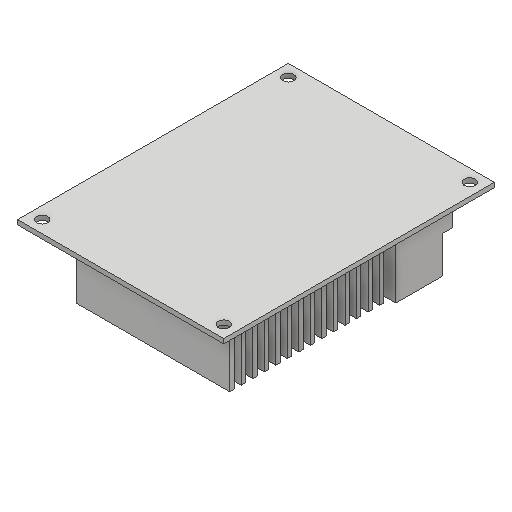
# Autodesk Inventor part: COTS_Generic_MKS_Mosfet_Module_For_Heatbed
Saved by Autodesk Inventor 2026.1 (Build 301233000, 233)
## iProperties
Created: 2017-07-26
Part Number: COTS_Generic_MKS_Mosfet_Module_For_Heatbed
Material: Ogólny
Document SubType Name: Modeling
Designer: Andrzej
Density: 1 g/cm^3
Appearance: Default
Author: Andrzej
Autodesk Inventor part; units mm, degrees
ref_plane "YZ Plane" through (0, 0, 0) normal (1, 0, 0) x (0, 1, 0)
ref_plane "XZ Plane" through (0, 0, 0) normal (0, 1, 0) x (-1, 0, 0)
ref_plane "XY Plane" through (0, 0, 0) normal (0, 0, 1) x (1, 0, 0)
sketch "Szkic1" plane through (0, 0, 0) normal (0, 0, 1) x (1, 0, 0)
  line L0 (-37.6373, 46.6232) -> (29.3627, 46.6232)
  line L1 (29.3627, 46.6232) -> (29.3627, -41.3768)
  line L2 (29.3627, -41.3768) -> (-37.6373, -41.3768)
  line L3 (-37.6373, -41.3768) -> (-37.6373, 46.6232)
  point P0 (0, 0)
  point P1 (-33.6373, 42.6232)
  point P2 (25.3627, 42.6232)
  point P3 (25.3627, -37.3768)
  point P4 (-33.6373, -37.3768)
  dimension "d0" = 88
  dimension "d1" = 67
  dimension "d2" = 59
  dimension "d3" = 80
  dimension "d4" = 80
  dimension "d5" = 59
  dimension "d6" = 4
  dimension "d7" = 4
  dimension "d8" = 4
  dimension "d9" = 4
  dimension "d10" = 4
  dimension "d11" = 4
  dimension "d12" = 4
  constraints: 8 end point, 2 parallel, 1 horizontal, 1 perpendicular
  measures "d0" distance of L2.end L0.start
  measures "d1" distance of L0.start L0.end
  measures "d2" distance of point (25.363, 42.623) point (-33.637, 42.623)
  measures "d3" distance of point (25.363, -37.377) point (25.363, 42.623)
  measures "d4" distance of point (-33.637, 42.623) point (-33.637, -37.377)
  measures "d5" distance of point (25.363, -37.377) point (-33.637, -37.377)
  measures "d6" distance from line of point (-33.637, -37.377) L3
  measures "d7" distance from line of L2 point (-33.637, -37.377)
  measures "d8" distance from line of L3 point (-33.637, 42.623)
  measures "d9" distance from line of L2 point (25.363, -37.377)
  measures "d10" distance from line of L1 point (25.363, -37.377)
  measures "d11" distance from line of L0 point (25.363, 42.623)
  measures "d12" distance from line of L1 point (25.363, 42.623)
extrude "Wyciągnięcie proste1" add sketch "Szkic1" along normal blind 1.5
hole "Otwór1" at (-33.6373, 42.6232, 0) at (25.3627, 42.6232, 0) at (25.3627, -37.3768, 0) at (-33.6373, -37.3768, 0) direction (0, 0, 1) diameter 3.6 end through all
sketch "Szkic2" plane through (0, 0, 0) normal (0, 0, -1) x (-1, 0, 0)
  line L0 (-18.8627, 21.1232) -> (31.1373, 21.1232)
  line L1 (31.1373, 21.1232) -> (31.1373, -28.8768)
  line L2 (31.1373, -28.8768) -> (-18.8627, -28.8768)
  line L3 (-18.8627, -28.8768) -> (-18.8627, 21.1232)
  circle A0 centre (-25.3627, -37.3768) radius 1.8 projected
  circle A1 centre (33.6373, 42.6232) radius 1.8 projected
  circle A2 centre (-25.3627, 42.6232) radius 1.8 projected
  circle A3 centre (33.6373, -37.3768) radius 1.8 projected
  line L4 (37.6373, 46.6232) -> (-29.3627, 46.6232) projected
  line L5 (-29.3627, 46.6232) -> (-29.3627, -41.3768) projected
  line L6 (-29.3627, -41.3768) -> (37.6373, -41.3768) projected
  line L7 (37.6373, -41.3768) -> (37.6373, 46.6232) projected
  line L8 (-16.3627, 42.6232) -> (23.6373, 42.6232)
  line L9 (23.6373, 42.6232) -> (23.6373, 27.6232)
  line L10 (23.6373, 27.6232) -> (-16.3627, 27.6232)
  line L11 (-16.3627, 27.6232) -> (-16.3627, 42.6232)
  point P0 (0, 0)
  dimension "d22" = 50
  dimension "d23" = 50
  dimension "d24" = 6.5
  dimension "d25" = 12.5
  dimension "d26" = 40
  dimension "d27" = 15
  dimension "d28" = 13
  dimension "d29" = 4
  constraints: 16 end point, 4 parallel, 2 horizontal, 2 perpendicular
  measures "d22" distance of L1.end L2.end
  measures "d23" distance of L0.end L1.end
  measures "d24" distance between parallel lines of L7 L1
  measures "d25" distance between parallel lines of L6 L2
  measures "d26" distance of L9.end L10.end
  measures "d27" distance of L8.end L9.end
  measures "d28" distance between parallel lines of L5 L11
  measures "d29" distance between parallel lines of L4 L8
extrude "Wyciągnięcie proste2" add sketch "Szkic2" along normal blind 25 contours L0 L1 L2 L3
sketch "Szkic3" plane through (0, 0, -25) normal (0, 0, -1) x (-1, 0, 0)
  line L0 (31.1373, 21.1232) -> (-18.8627, 21.1232) projected
  line L1 (-18.8627, 21.1232) -> (-18.8627, -28.8768) projected
  line L2 (-18.8627, -28.8768) -> (31.1373, -28.8768) projected
  line L3 (31.1373, -28.8768) -> (31.1373, 21.1232) projected
  line L4 (-18.8627, -28.8768) -> (-18.8627, 21.1232) projected
  line L5 (-18.8627, -27.5268) -> (31.1373, -27.5268)
  line L6 (31.1373, -27.5268) -> (31.1373, -25.1768)
  line L7 (31.1373, -25.1768) -> (-18.8627, -25.1768)
  line L8 (-18.8627, -25.1768) -> (-18.8627, -27.5268)
  line L9 (-18.8627, -23.7768) -> (31.1373, -23.7768)
  line L10 (31.1373, -23.7768) -> (31.1373, -21.4268)
  line L11 (31.1373, -21.4268) -> (-18.8627, -21.4268)
  line L12 (-18.8627, -21.4268) -> (-18.8627, -23.7768)
  line L13 (-18.8627, -20.0268) -> (31.1373, -20.0268)
  line L14 (31.1373, -20.0268) -> (31.1373, -17.6768)
  line L15 (31.1373, -17.6768) -> (-18.8627, -17.6768)
  line L16 (-18.8627, -17.6768) -> (-18.8627, -20.0268)
  line L17 (-18.8627, -16.2768) -> (31.1373, -16.2768)
  line L18 (31.1373, -16.2768) -> (31.1373, -13.9268)
  line L19 (31.1373, -13.9268) -> (-18.8627, -13.9268)
  line L20 (-18.8627, -13.9268) -> (-18.8627, -16.2768)
  line L21 (-18.8627, -12.5268) -> (31.1373, -12.5268)
  line L22 (31.1373, -12.5268) -> (31.1373, -10.1768)
  line L23 (31.1373, -10.1768) -> (-18.8627, -10.1768)
  line L24 (-18.8627, -10.1768) -> (-18.8627, -12.5268)
  line L25 (-18.8627, -8.7768) -> (31.1373, -8.7768)
  line L26 (31.1373, -8.7768) -> (31.1373, -6.4268)
  line L27 (31.1373, -6.4268) -> (-18.8627, -6.4268)
  line L28 (-18.8627, -6.4268) -> (-18.8627, -8.7768)
  line L29 (-18.8627, -5.0268) -> (31.1373, -5.0268)
  line L30 (31.1373, -5.0268) -> (31.1373, -2.6768)
  line L31 (31.1373, -2.6768) -> (-18.8627, -2.6768)
  line L32 (-18.8627, -2.6768) -> (-18.8627, -5.0268)
  line L33 (-18.8627, -1.2768) -> (31.1373, -1.2768)
  line L34 (31.1373, -1.2768) -> (31.1373, 1.0732)
  line L35 (31.1373, 1.0732) -> (-18.8627, 1.0732)
  line L36 (-18.8627, 1.0732) -> (-18.8627, -1.2768)
  line L37 (-18.8627, 2.4732) -> (31.1373, 2.4732)
  line L38 (31.1373, 2.4732) -> (31.1373, 4.8232)
  line L39 (31.1373, 4.8232) -> (-18.8627, 4.8232)
  line L40 (-18.8627, 4.8232) -> (-18.8627, 2.4732)
  line L41 (-18.8627, 6.2232) -> (31.1373, 6.2232)
  line L42 (31.1373, 6.2232) -> (31.1373, 8.5732)
  line L43 (31.1373, 8.5732) -> (-18.8627, 8.5732)
  line L44 (-18.8627, 8.5732) -> (-18.8627, 6.2232)
  line L45 (-18.8627, 9.9732) -> (31.1373, 9.9732)
  line L46 (31.1373, 9.9732) -> (31.1373, 12.3232)
  line L47 (31.1373, 12.3232) -> (-18.8627, 12.3232)
  line L48 (-18.8627, 12.3232) -> (-18.8627, 9.9732)
  line L49 (-18.8627, 13.7232) -> (31.1373, 13.7232)
  line L50 (31.1373, 13.7232) -> (31.1373, 16.0732)
  line L51 (31.1373, 16.0732) -> (-18.8627, 16.0732)
  line L52 (-18.8627, 16.0732) -> (-18.8627, 13.7232)
  line L53 (-18.8627, 17.4732) -> (31.1373, 17.4732)
  line L54 (31.1373, 17.4732) -> (31.1373, 19.8232)
  line L55 (31.1373, 19.8232) -> (-18.8627, 19.8232)
  line L56 (-18.8627, 19.8232) -> (-18.8627, 17.4732)
  point P0 (0, 0)
  dimension "d32" = 50
  dimension "d33" = 2.35
  dimension "d34" = 1.35
  dimension "d37" = 3.75
  constraints: 104 end point, 2 parallel, 1 horizontal, 1 perpendicular, 1 point on line, 1 vertical, 96 other
  measures "d32" distance of L7.end L6.end
  measures "d33" distance of L6.end L5.end
  measures "d34" distance between parallel lines of L2 L5
  measures "d37" distance of L5.start L9.start
extrude "Wyciągnięcie proste3" cut sketch "Szkic3" against normal blind 17 contours L3 L53 L1 L55 | L3 L49 L1 L51 | L3 L45 L1 L47 | L3 L41 L1 L43 | L3 L37 L1 L39 | L3 L33 L1 L35 | L3 L29 L1 L31 | L3 L25 L1 L27 | L3 L21 L1 L23 | L3 L17 L1 L19 | L3 L13 L1 L15 | L3 L9 L1 L11 | L3 L5 L1 L7
sketch "Szkic4" plane through (-31.1373, -28.8768, 0) normal (-1, 0, 0) x (0, 0, 1)
  line L0 (-8, 42.6) -> (-25, 42.6) projected
  line L1 (-25, 41.2) -> (-25, 42.6) projected
  line L2 (-25, 41.2) -> (-8, 41.2) projected
  line L3 (-8, 41.2) -> (-8, 38.85) projected
  line L4 (-8, 38.85) -> (-25, 38.85) projected
  line L5 (-25, 37.45) -> (-25, 38.85) projected
  line L6 (-25, 37.45) -> (-8, 37.45) projected
  line L7 (-8, 37.45) -> (-8, 35.1) projected
  line L8 (-8, 35.1) -> (-25, 35.1) projected
  line L9 (-25, 33.7) -> (-25, 35.1) projected
  line L10 (-25, 33.7) -> (-8, 33.7) projected
  line L11 (-8, 33.7) -> (-8, 31.35) projected
  line L12 (-8, 31.35) -> (-25, 31.35) projected
  line L13 (-25, 29.95) -> (-25, 31.35) projected
  line L14 (-25, 29.95) -> (-8, 29.95) projected
  line L15 (-8, 29.95) -> (-8, 27.6) projected
  line L16 (-8, 27.6) -> (-25, 27.6) projected
  line L17 (-25, 26.2) -> (-25, 27.6) projected
  line L18 (-25, 26.2) -> (-8, 26.2) projected
  line L19 (-8, 26.2) -> (-8, 23.85) projected
  line L20 (-8, 23.85) -> (-25, 23.85) projected
  line L21 (-25, 22.45) -> (-25, 23.85) projected
  line L22 (-25, 22.45) -> (-8, 22.45) projected
  line L23 (-8, 22.45) -> (-8, 20.1) projected
  line L24 (-8, 20.1) -> (-25, 20.1) projected
  line L25 (-25, 18.7) -> (-25, 20.1) projected
  line L26 (-25, 18.7) -> (-8, 18.7) projected
  line L27 (-8, 18.7) -> (-8, 16.35) projected
  line L28 (-8, 16.35) -> (-25, 16.35) projected
  line L29 (-25, 14.95) -> (-25, 16.35) projected
  line L30 (-25, 14.95) -> (-8, 14.95) projected
  line L31 (-8, 14.95) -> (-8, 12.6) projected
  line L32 (-8, 12.6) -> (-25, 12.6) projected
  line L33 (-25, 11.2) -> (-25, 12.6) projected
  line L34 (-25, 11.2) -> (-8, 11.2) projected
  line L35 (-8, 11.2) -> (-8, 8.85) projected
  line L36 (-8, 8.85) -> (-25, 8.85) projected
  line L37 (-25, 7.45) -> (-25, 8.85) projected
  line L38 (-25, 7.45) -> (-8, 7.45) projected
  line L39 (-8, 7.45) -> (-8, 5.1) projected
  line L40 (-8, 5.1) -> (-25, 5.1) projected
  line L41 (-25, 3.7) -> (-25, 5.1) projected
  line L42 (-25, 3.7) -> (-8, 3.7) projected
  line L43 (-8, 3.7) -> (-8, 1.35) projected
  line L44 (-8, 1.35) -> (-25, 1.35) projected
  line L45 (-25, 0) -> (-25, 1.35) projected
  line L46 (0, 0) -> (-25, 0) projected
  line L47 (0, 50) -> (0, 0) projected
  line L48 (0, 50) -> (-25, 50) projected
  line L49 (-25, 48.7) -> (-25, 50) projected
  line L50 (-25, 48.7) -> (-8, 48.7) projected
  line L51 (-8, 48.7) -> (-8, 46.35) projected
  line L52 (-8, 46.35) -> (-25, 46.35) projected
  line L53 (-25, 44.95) -> (-25, 46.35) projected
  line L54 (-25, 44.95) -> (-8, 44.95) projected
  line L55 (-8, 44.95) -> (-8, 42.6) projected
  line L56 (0, 50) -> (0, 0) projected
  line L57 (0, 50) -> (-25, 50) projected
  line L58 (0, 0) -> (-5, 0)
  line L59 (-5, 0) -> (-5, 50)
  line L60 (-5, 50) -> (0, 50)
  line L61 (0, 50) -> (0, 0)
  point P0 (0, 28.8768)
  dimension "d44" = 5
  constraints: 8 end point, 2 parallel, 1 horizontal, 1 perpendicular, 1 point on line
  measures "d44" distance of L59.end L60.end
extrude "Wyciągnięcie proste4" cut sketch "Szkic4" against normal blind 16 contours L48 L47 L46 L59
sketch "Szkic5" plane through (18.8627, -28.8768, 0) normal (1, 0, 0) x (0, 0, -1)
  line L0 (25, 42.6) -> (8, 42.6) projected
  line L1 (8, 42.6) -> (8, 44.95) projected
  line L2 (8, 44.95) -> (25, 44.95) projected
  line L3 (25, 46.35) -> (25, 44.95) projected
  line L4 (25, 46.35) -> (8, 46.35) projected
  line L5 (8, 46.35) -> (8, 48.7) projected
  line L6 (8, 48.7) -> (25, 48.7) projected
  line L7 (25, 50) -> (25, 48.7) projected
  line L8 (0, 50) -> (25, 50) projected
  line L9 (0, 0) -> (0, 50) projected
  line L10 (0, 0) -> (25, 0) projected
  line L11 (25, 1.35) -> (25, 0) projected
  line L12 (25, 1.35) -> (8, 1.35) projected
  line L13 (8, 1.35) -> (8, 3.7) projected
  line L14 (8, 3.7) -> (25, 3.7) projected
  line L15 (25, 5.1) -> (25, 3.7) projected
  line L16 (25, 5.1) -> (8, 5.1) projected
  line L17 (8, 5.1) -> (8, 7.45) projected
  line L18 (8, 7.45) -> (25, 7.45) projected
  line L19 (25, 8.85) -> (25, 7.45) projected
  line L20 (25, 8.85) -> (8, 8.85) projected
  line L21 (8, 8.85) -> (8, 11.2) projected
  line L22 (8, 11.2) -> (25, 11.2) projected
  line L23 (25, 12.6) -> (25, 11.2) projected
  line L24 (25, 12.6) -> (8, 12.6) projected
  line L25 (8, 12.6) -> (8, 14.95) projected
  line L26 (8, 14.95) -> (25, 14.95) projected
  line L27 (25, 16.35) -> (25, 14.95) projected
  line L28 (25, 16.35) -> (8, 16.35) projected
  line L29 (8, 16.35) -> (8, 18.7) projected
  line L30 (8, 18.7) -> (25, 18.7) projected
  line L31 (25, 20.1) -> (25, 18.7) projected
  line L32 (25, 20.1) -> (8, 20.1) projected
  line L33 (8, 20.1) -> (8, 22.45) projected
  line L34 (8, 22.45) -> (25, 22.45) projected
  line L35 (25, 23.85) -> (25, 22.45) projected
  line L36 (25, 23.85) -> (8, 23.85) projected
  line L37 (8, 23.85) -> (8, 26.2) projected
  line L38 (8, 26.2) -> (25, 26.2) projected
  line L39 (25, 27.6) -> (25, 26.2) projected
  line L40 (25, 27.6) -> (8, 27.6) projected
  line L41 (8, 27.6) -> (8, 29.95) projected
  line L42 (8, 29.95) -> (25, 29.95) projected
  line L43 (25, 31.35) -> (25, 29.95) projected
  line L44 (25, 31.35) -> (8, 31.35) projected
  line L45 (8, 31.35) -> (8, 33.7) projected
  line L46 (8, 33.7) -> (25, 33.7) projected
  line L47 (25, 35.1) -> (25, 33.7) projected
  line L48 (25, 35.1) -> (8, 35.1) projected
  line L49 (8, 35.1) -> (8, 37.45) projected
  line L50 (8, 37.45) -> (25, 37.45) projected
  line L51 (25, 38.85) -> (25, 37.45) projected
  line L52 (25, 38.85) -> (8, 38.85) projected
  line L53 (8, 38.85) -> (8, 41.2) projected
  line L54 (8, 41.2) -> (25, 41.2) projected
  line L55 (25, 42.6) -> (25, 41.2) projected
  line L56 (5, 0) -> (5, 50) projected
  point P0 (0, 28.8768)
extrude "Wyciągnięcie proste5" cut sketch "Szkic5" against normal blind 16 contours L56 L10 L9 L8
sketch "Szkic6" plane through (-31.1373, 21.1232, -25) normal (0, 1, 0) x (1, 0, 0)
  line L0 (34, -25) -> (34, -20) projected
  line L1 (34, -20) -> (50, -20) projected
  line L2 (50, -20) -> (50, 0) projected
  line L3 (0, 0) -> (50, 0) projected
  line L4 (0, -20) -> (0, 0) projected
  line L5 (0, -20) -> (16, -20) projected
  line L6 (16, -20) -> (16, -25) projected
  line L7 (34, -25) -> (16, -25) projected
  line L8 (16, -25) -> (16, -20) projected
  line L9 (34, -20) -> (50, -20) projected
  line L10 (16, -25) -> (34, -25)
  line L11 (34, -25) -> (34, -20)
  line L12 (34, -20) -> (16, -20)
  line L13 (16, -20) -> (16, -25)
  point P0 (31.1373, -25)
  constraints: 8 end point, 2 parallel, 1 horizontal, 1 perpendicular
extrude "Wyciągnięcie proste6" cut sketch "Szkic6" against normal blind 12 contours L7 L6 L12 L0
sketch "Szkic7" plane through (-31.1373, -28.8768, -25) normal (0, -1, 0) x (1, 0, 0)
  line L0 (34, 20) -> (34, 25) projected
  line L1 (16, 25) -> (34, 25) projected
  line L2 (16, 25) -> (16, 20) projected
  line L3 (16, 20) -> (0, 20) projected
  line L4 (0, 20) -> (0, 0) projected
  line L5 (50, 0) -> (0, 0) projected
  line L6 (50, 20) -> (50, 0) projected
  line L7 (50, 20) -> (34, 20) projected
  line L8 (16, 20) -> (34, 20) projected
  point P0 (31.1373, 25)
extrude "Wyciągnięcie proste7" cut sketch "Szkic7" against normal blind 12 contours L8 L2 L1 L0
extrude "Wyciągnięcie proste8" add sketch "Szkic2" along normal blind 4.5 contours L8 L9 L10 L11
sketch "Szkic8" plane through (0, 0, -4.5) normal (0, 0, -1) x (-1, 0, 0)
  line L0 (23.6373, 42.6232) -> (-16.3627, 42.6232) projected
  line L1 (-16.3627, 42.6232) -> (-16.3627, 27.6232) projected
  line L2 (-16.3627, 27.6232) -> (23.6373, 27.6232) projected
  line L3 (23.6373, 27.6232) -> (23.6373, 42.6232) projected
  line L4 (-16.3627, 27.6232) -> (23.6373, 27.6232)
  line L5 (23.6373, 27.6232) -> (23.6373, 46.1232)
  line L6 (23.6373, 46.1232) -> (-16.3627, 46.1232)
  line L7 (-16.3627, 46.1232) -> (-16.3627, 27.6232)
  point P0 (0, 0)
  dimension "d55" = 40
  dimension "d56" = 18.5
  constraints: 8 end point, 2 parallel, 1 horizontal, 1 perpendicular
  measures "d55" distance of L6.end L5.end
  measures "d56" distance of L5.end L4.end
extrude "Wyciągnięcie proste9" add sketch "Szkic8" along normal blind 13
sketch "Szkic9" plane through (0, 0, -17.5) normal (0, 0, -1) x (-1, 0, 0)
  line L0 (-16.3627, 27.6232) -> (23.6373, 27.6232) projected
  line L1 (23.6373, 27.6232) -> (23.6373, 46.1232) projected
  line L2 (23.6373, 46.1232) -> (-16.3627, 46.1232) projected
  line L3 (-16.3627, 46.1232) -> (-16.3627, 27.6232) projected
  line L4 (23.6373, 42.6232) -> (-16.3627, 42.6232) projected
  point P0 (0, 0)
extrude "Wyciągnięcie proste10" add sketch "Szkic9" along normal blind 12 contours L3 L4 L1 L0
sketch "Szkic10" plane through (0, 0, -29.5) normal (0, 0, -1) x (-1, 0, 0)
  line L0 (-16.3627, 27.6232) -> (23.6373, 27.6232) projected
  line L1 (23.6373, 27.6232) -> (23.6373, 42.6232) projected
  line L2 (23.6373, 42.6232) -> (-16.3627, 42.6232) projected
  line L3 (-16.3627, 42.6232) -> (-16.3627, 27.6232) projected
  point P0 (0, 0)
  point P1 (18.7191, 35.1232)
  point P2 (8.7191, 35.1232)
  point P3 (-1.2809, 35.1232)
  point P4 (-11.2809, 35.1232)
  dimension "d61" = 15
  dimension "d62" = 7.5
  dimension "d63" = 7.5
  dimension "d64" = 7.5
  dimension "d65" = 7.5
  dimension "d66" = 10
  dimension "d67" = 10
  dimension "d68" = 10
  measures "d61" distance of L0.end L1.end
  measures "d62" distance from line of L0 point (18.719, 35.123)
  measures "d63" distance from line of L0 point (8.719, 35.123)
  measures "d64" distance from line of L0 point (-1.281, 35.123)
  measures "d65" distance from line of L0 point (-11.281, 35.123)
  measures "d66" distance of point (8.719, 35.123) point (18.719, 35.123)
  measures "d67" distance of point (-1.281, 35.123) point (8.719, 35.123)
  measures "d68" distance of point (-1.281, 35.123) point (-11.281, 35.123)
hole "Otwór2" at (-18.7191, 35.1232, -29.5) at (-8.7191, 35.1232, -29.5) at (1.2809, 35.1232, -29.5) at (11.2809, 35.1232, -29.5) direction (0, 0, 1) diameter 6.4 depth 3.6
equation "\"d4\" = d3"
equation "\"d5\" = d2"
equation "\"d6\" = -0.5 * d5 + 0.5 * d1"
equation "\"d7\" = -0.5 * d4 + 0.5 * d0"
equation "\"d8\" = d6"
equation "\"d9\" = d7"
equation "\"d64\" = d62"
equation "\"d67\" = d66"
equation "\"d68\" = d66"
